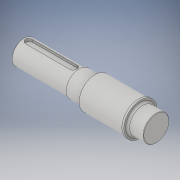
# Autodesk Inventor part: GonjenoVratilo
Saved by Autodesk Inventor 2018 (Build 220112000, 112)
## iProperties
Created: 2018-11-17
Part Number: GonjenoVratilo
Material: Generic
Document SubType Name: Modeling
Designer: Kristijan
Density: 1 g/cm^3
Appearance: Default
Author: Kristijan
Autodesk Inventor part; units mm, degrees
ref_plane "YZ Plane" through (0, 0, 0) normal (1, 0, 0) x (0, 1, 0)
ref_plane "XY Plane" through (0, 0, 0) normal (0, 0, 1) x (1, 0, 0)
sketch "Sketch1" plane through (0, 0, 0) normal (0, 0, 1) x (1, 0, 0)
  point P0 (0, 0)
sketch "Sketch2" plane through (0, 0, 0) normal (0, 0, 1) x (1, 0, 0)
  line L0 (0, 0) -> (0, 29)
  line L1 (1, 30) -> (140, 30)
  line L2 (140, 30) -> (140, 32.5)
  line L3 (140, 32.5) -> (175, 32.5)
  line L4 (180, 37.5) -> (180, 40)
  line L5 (180, 40) -> (290, 40)
  line L6 (290, 40) -> (290, 42)
  line L7 (290, 42) -> (295, 42)
  line L8 (295, 42) -> (295, 37.5)
  line L9 (300, 32.5) -> (334, 32.5)
  line L10 (335, 31.5) -> (335, 0)
  line L11 (335, 0) -> (0, 0)
  line L12 (0, 29) -> (1, 30)
  line L13 (334, 32.5) -> (335, 31.5)
  arc A0 (175, 32.5) -> (180, 37.5) centre (175, 37.5) ccw
  arc A1 (295, 37.5) -> (300, 32.5) centre (300, 37.5) ccw
  line L14 (-67, 0) -> (402, 0) projected
  point P0 (0, 30)
  point P1 (180, 32.5)
  point P2 (295, 32.5)
  point P3 (335, 32.5)
  dimension "d0" = 30
  dimension "d1" = 140
  dimension "d2" = 32.5
  dimension "d3" = 40
  dimension "d4" = 110
  dimension "d5" = 5
  dimension "d6" = 40
  dimension "d7" = 32.5
  dimension "d8" = 40
  dimension "d9" = 2
  dimension "d10" = 1
  dimension "d11" = 45
  dimension "d12" = 1
  dimension "d13" = 45
  dimension "d14" = 5
  constraints: 28 end point, 10 perpendicular, 8 point on line, 4 point on circle, 4 tangent, 2 centre point, 2 vertical, 1 equal radius
  measures "d0" distance between parallel lines of L11 L1
  measures "d1" distance of point (0, 30) L1.end
  measures "d2" distance between parallel lines of L11 L3
  measures "d3" distance of L2.end point (180, 32.5)
  measures "d4" distance of L4.end L5.end
  measures "d5" distance of L6.end L7.end
  measures "d6" distance of point (295, 32.5) point (335, 32.5)
  measures "d7" distance between parallel lines of L11 L9
  measures "d8" distance between parallel lines of L11 L5
  measures "d9" distance of L5.end L6.end
  measures "d10" distance of L0.end point (0, 30)
  measures "d11" angle of L0 L12
  measures "d12" distance of L9.end point (335, 32.5)
  measures "d13" angle of L9 L13
  measures "d14" radius of A0
revolve "Revolution1" add sketch "Sketch2" angle 360 about axis through (-10, 0, 0) along (1, 0, 0)
ref_plane "Work Plane1" through (70.5, 30, 0) normal (0, 1, 0) x (-1, 0, 0)
ref_plane "Work Plane2" through (235, 40, 0) normal (0, 1, 0) x (-1, 0, 0)
sketch "Sketch3" plane through (70.5, 30, 0) normal (0, 1, 0) x (-1, 0, 0)
  line L0 (56.5, 0) -> (-55.5, 0) construction
  line L1 (56.5, 9) -> (-55.5, 9)
  line L2 (-55.5, -9) -> (56.5, -9)
  arc A0 (56.5, -9) -> (56.5, 9) centre (56.5, 0) ccw
  arc A1 (-55.5, 9) -> (-55.5, -9) centre (-55.5, 0) ccw
  line L3 (-69.5, 32.5) -> (-69.5, -32.5) projected
  point P0 (70.5, 0)
  point P1 (0.5, 0)
  dimension "d16" = 130
  dimension "d17" = 5
  dimension "d18" = 9
  constraints: 8 end point, 4 point on circle, 4 tangent, 2 centre point, 1 horizontal, 1 midpoint, 1 parallel
  measures "d17" distance edge to line of A1 L3
  measures "d18" radius of A0
extrude "Extrusion1" cut sketch "Sketch3" against normal blind 7
equation "\"d6\" = d3"
equation "\"d7\" = d2"
equation "\"d12\" = d10"
equation "\"d13\" = d11"
body "Solid1"
